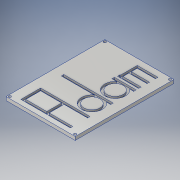
# Autodesk Inventor part: Adam Name Plate
Saved by Autodesk Inventor 2016 (Build 200138000, 138)
## iProperties
Created: 2016-09-22
Part Number: Adam Name Plate
Material: Aluminum
Document SubType Name: Modeling
Designer: Adam Popescu
Density: 2.7 g/cm^3
Appearance: Aluminum - Flat
Sheet Metal Rule: Default
Author: Adam Popescu
Autodesk Inventor part; units mm, degrees
ref_plane "YZ Plane" through (0, 0, 0) normal (1, 0, 0) x (0, 1, 0)
ref_plane "XZ Plane" through (0, 0, 0) normal (0, 1, 0) x (-1, 0, 0)
ref_plane "XY Plane" through (0, 0, 0) normal (0, 0, 1) x (1, 0, 0)
sketch "Sketch1" plane through (0, 0, 0) normal (0, 1, 0) x (-1, 0, 0)
  line L0 (121.4597, 127.3409) -> (-56.3403, 127.3409)
  line L1 (-56.3403, 127.3409) -> (-56.3403, -126.6591)
  line L2 (-56.3403, -126.6591) -> (121.4597, -126.6591)
  line L3 (121.4597, -126.6591) -> (121.4597, 127.3409)
  point P0 (0, 0)
  dimension "d0" = 254
  dimension "d1" = 177.8
  constraints: 8 end point, 2 parallel, 1 horizontal, 1 perpendicular
  measures "d0" distance of L2.end L0.start
  measures "d1" distance of L0.start L0.end
sketch "Sketch2" plane through (0, 0, 0) normal (0, 1, 0) x (-1, 0, 0)
  point P0 (0, 0)
extrude "Extrusion1" add sketch "Sketch1" along normal blind 8.89
sketch "Sketch3" plane through (0, 8.89, 0) normal (0, 1, 0) x (1, 0, 0)
  line L0 (30.9403, -114.6409) -> (30.9403, -108.2909)
  line L1 (-121.4597, -127.3409) -> (56.3403, -127.3409) projected
  line L2 (56.3403, -127.3409) -> (56.3403, 126.6591) projected
  line L3 (30.9403, -108.2909) -> (-96.0597, -108.2909)
  line L4 (-96.0597, -108.2909) -> (-96.0597, -114.6409)
  line L5 (-96.0597, -114.6409) -> (30.9403, -114.6409)
  line L6 (-121.4597, 126.6591) -> (-121.4597, -127.3409) projected
  line L7 (-96.0597, -108.2909) -> (-89.7097, -108.2909)
  line L8 (-89.7097, -108.2909) -> (-89.7097, -63.8409)
  line L9 (-89.7097, -63.8409) -> (-96.0597, -63.8409)
  line L10 (-96.0597, -63.8409) -> (-96.0597, -108.2909)
  line L11 (-96.0597, -63.8409) -> (30.9403, -63.8409)
  line L12 (30.9403, -63.8409) -> (30.9403, -70.1909)
  line L13 (30.9403, -70.1909) -> (-96.0597, -70.1909)
  line L14 (-96.0597, -70.1909) -> (-96.0597, -63.8409)
  line L15 (-35.7347, -114.6409) -> (-29.3847, -114.6409)
  line L16 (-29.3847, -114.6409) -> (-29.3847, -63.8409)
  line L17 (-29.3847, -63.8409) -> (-35.7347, -63.8409)
  line L18 (-35.7347, -63.8409) -> (-35.7347, -114.6409)
  point P0 (0, 0)
  dimension "d4" = 6.35
  dimension "d5" = 12.7
  dimension "d6" = 25.4
  dimension "d7" = 25.4
  dimension "d8" = 6.35
  dimension "d10" = 127
  dimension "d11" = 6.35
  dimension "d12" = 50.8
  dimension "d13" = 6.35
  dimension "d14" = 60.325
  dimension "d15" = 60.325
  constraints: 32 end point, 6 parallel, 5 perpendicular, 4 horizontal, 2 point on line, 1 vertical
  measures "d4" distance of L0.start L0.end
  measures "d5" distance from line of L1 L0.start
  measures "d6" distance between parallel lines of L2 L0
  measures "d7" distance between parallel lines of L4 L6
  measures "d8" distance of L8.end L9.end
  measures "d10" distance of L9.end L11.end
  measures "d11" distance between parallel lines of L11 L13
  measures "d12" distance between parallel lines of L9 L5
  measures "d13" distance between parallel lines of L16 L18
  measures "d14" distance between parallel lines of L10 L18
  measures "d15" distance between parallel lines of L0 L16
sketch "Sketch4" plane through (0, 8.89, 0) normal (0, 1, 0) x (1, 0, 0)
  point P0 (0, 0)
extrude "Extrusion2" cut sketch "Sketch3" against normal blind 5.08 contours L5 L16 L3 L0 | L5 L18 L3 L16 | L3 L18 L13 L16 | L5 L4 L3 L18 | L16 L11 L12 L13 | L13 L18 L11 L16 | L3 L10 L13 L8 | L13 L8 L11 L18 | L13 L10 L9 L8
sketch "Sketch5" plane through (0, 8.89, 0) normal (0, 1, 0) x (1, 0, 0)
  line L0 (-96.0597, -4.1509) -> (30.9403, -4.1509)
  line L1 (30.9403, -4.1509) -> (30.9403, -10.5009)
  line L2 (30.9403, -10.5009) -> (-96.0597, -10.5009)
  line L3 (-96.0597, -10.5009) -> (-96.0597, -4.1509)
  line L4 (-96.0597, -63.8409) -> (30.9403, -63.8409) projected
  line L5 (-121.4597, 126.6591) -> (-121.4597, -127.3409) projected
  circle A0 centre (4.1687, -32.0909) radius 20.4377
  circle A1 centre (4.1687, -32.0909) radius 26.7877
  line L6 (56.3403, -127.3409) -> (56.3403, 126.6591) projected
  point P0 (0, 0)
  dimension "d18" = 53.34
  dimension "d19" = 6.35
  dimension "d20" = 127
  dimension "d21" = 25.4
  dimension "d22" = 6.35
  dimension "d23" = 21.59
  dimension "d24" = 100.2284
  dimension "d25" = 52.1716
  constraints: 8 end point, 2 centre point, 2 parallel, 1 coincident, 1 horizontal, 1 perpendicular
  measures "d18" distance between parallel lines of L4 L2
  measures "d19" distance of L2.end L0.start
  measures "d20" distance of L1.end L2.end
  measures "d21" distance between parallel lines of L5 L3
  measures "d22" radial gap between concentric circles of A1 A0
  measures "d23" distance from line of L2 A1.centre
  measures "d24" distance from line of L3 A1.centre
  measures "d25" distance from line of L6 A1.centre
sketch "Sketch6" plane through (0, 8.89, 0) normal (0, 1, 0) x (1, 0, 0)
  point P0 (0, 0)
extrude "Extrusion3" cut sketch "Sketch5" against normal blind 5.08
sketch "Sketch7" plane through (0, 8.89, 0) normal (0, 1, 0) x (1, 0, 0)
  line L0 (30.9403, 55.5391) -> (-32.5597, 55.5391)
  line L1 (-32.5597, 55.5391) -> (-32.5597, 48.0334)
  line L2 (-32.5597, 48.0334) -> (30.9403, 48.0334)
  line L3 (30.9403, 48.0334) -> (30.9403, 55.5391)
  line L4 (56.3403, -127.3409) -> (56.3403, 126.6591) projected
  line L5 (30.9403, -4.1509) -> (30.9403, -10.5009) projected
  circle A0 centre (4.1687, 27.5991) radius 20.4343
  circle A1 centre (4.1687, 27.5991) radius 26.7843
  line L6 (-96.0597, -4.1509) -> (30.9403, -4.1509) projected
  line L7 (-96.0597, -63.8409) -> (30.9403, -63.8409) projected
  arc A2 (-11.6885, -10.5009) -> (20.0259, -10.5009) centre (4.1687, -32.0909) ccw projected
  point P0 (0, 0)
  dimension "d31" = 25.4
  dimension "d35" = 31.75
  dimension "d37" = 27.94
  dimension "d39" = 27.94
  dimension "d40" = 63.5
  dimension "d42" = 25.4
  dimension "d43" = 26.7716
  dimension "d44" = 26.7716
  dimension "d45" = 31.75
  dimension "d46" = 6.35
  constraints: 8 end point, 2 centre point, 2 parallel, 1 coincident, 1 horizontal, 1 perpendicular, 1 tangent
  measures "d31" distance between parallel lines of L4 L5
  measures "d35" distance from line of L7 A2.centre
  measures "d37" distance from line of L6 A2.centre
  measures "d39" distance from line of L0 A0.centre
  measures "d40" distance between parallel lines of L3 L1
  measures "d42" distance between parallel lines of L4 L3
  measures "d43" distance from line of L3 A0.centre
  measures "d44" distance from line of L5 A2.centre
  measures "d45" distance from line of L6 A0.centre
  measures "d46" radial gap between concentric circles of A0 A1
sketch "Sketch9" plane through (0, 8.89, 0) normal (0, 1, 0) x (1, 0, 0)
  point P0 (0, 0)
extrude "Extrusion4" cut sketch "Sketch7" against normal blind 5.08 contours A1 L2 | L2 A1
sketch "Sketch12" plane through (0, 8.89, 0) normal (0, 1, 0) x (1, 0, 0)
  point P0 (0, 0)
sketch "Sketch13" plane through (0, 8.89, 0) normal (0, 1, 0) x (1, 0, 0)
  line L0 (30.9403, 48.4271) -> (-24.9397, 48.4271)
  line L1 (-24.9397, 48.4271) -> (-24.9397, 54.7771)
  line L2 (-24.9397, 54.7771) -> (30.9403, 54.7771)
  line L3 (30.9403, 54.7771) -> (30.9403, 48.4271)
  line L4 (56.3403, -127.3409) -> (56.3403, 126.6591) projected
  line L5 (-96.0597, -4.1509) -> (30.9403, -4.1509) projected
  point P0 (0, 0)
  dimension "d53" = 6.35
  dimension "d54" = 25.4
  dimension "d55" = 55.88
  dimension "d56" = 52.578
  constraints: 8 end point, 2 parallel, 1 horizontal, 1 perpendicular
  measures "d53" distance of L0.end L1.end
  measures "d54" distance between parallel lines of L4 L3
  measures "d55" distance of L0.start L0.end
  measures "d56" distance between parallel lines of L5 L0
extrude "Extrusion5" cut sketch "Sketch13" against normal blind 5.08
sketch "Sketch15" plane through (0, 8.89, 0) normal (0, 1, 0) x (1, 0, 0)
  point P0 (0, 0)
sketch "Sketch16" plane through (0, 8.89, 0) normal (0, 1, 0) x (1, 0, 0)
  point P0 (0, 0)
sketch "Sketch14" plane through (0, 8.89, 0) normal (0, 1, 0) x (1, 0, 0)
  line L0 (30.9403, 61.1271) -> (-23.4198, 61.1271)
  line L1 (-23.4198, 61.1271) -> (-23.4198, 67.4771)
  line L2 (-23.4198, 67.4771) -> (30.9403, 67.4771)
  line L3 (30.9403, 67.4771) -> (30.9403, 61.1271)
  line L4 (-24.9397, 54.7771) -> (30.9403, 54.7771) projected
  line L5 (-22.0163, 67.4771) -> (-15.6663, 67.4771)
  line L6 (-15.6663, 67.4771) -> (-15.6663, 82.7171)
  line L7 (-15.6663, 82.7171) -> (-22.0163, 82.7171)
  line L8 (-22.0163, 82.7171) -> (-22.0163, 67.4771)
  line L9 (-22.0163, 82.7171) -> (30.9403, 82.7171)
  line L10 (30.9403, 82.7171) -> (30.9403, 89.0671)
  line L11 (30.9403, 89.0671) -> (-22.0163, 89.0671)
  line L12 (-22.0163, 89.0671) -> (-22.0163, 82.7171)
  line L13 (-22.0163, 89.0671) -> (-15.6663, 89.0671)
  line L14 (-15.6663, 89.0671) -> (-15.6663, 104.3071)
  line L15 (-15.6663, 104.3071) -> (-22.0163, 104.3071)
  line L16 (-22.0163, 104.3071) -> (-22.0163, 89.0671)
  line L17 (-22.0163, 104.3071) -> (30.9403, 104.3071)
  line L18 (30.9403, 104.3071) -> (30.9403, 110.6571)
  line L19 (30.9403, 110.6571) -> (-22.0163, 110.6571)
  line L20 (-22.0163, 110.6571) -> (-22.0163, 104.3071)
  point P0 (0, 0)
  dimension "d59" = 6.35
  dimension "d60" = 6.35
  dimension "d61" = 6.35
  dimension "d62" = 15.24
  dimension "d63" = 6.35
  dimension "d64" = 15.24
  dimension "d65" = 6.35
  dimension "d66" = 6.35
  constraints: 40 end point, 10 parallel, 5 horizontal, 5 perpendicular, 1 point on line
  measures "d59" distance between parallel lines of L4 L0
  measures "d60" distance between parallel lines of L2 L0
  measures "d61" distance between parallel lines of L6 L8
  measures "d62" distance of L7.end L5.start
  measures "d63" distance between parallel lines of L11 L9
  measures "d64" distance of L15.end L11.end
  measures "d65" distance of L14.end L15.end
  measures "d66" distance of L17.end L18.end
extrude "Extrusion6" cut sketch "Sketch14" against normal blind 5.08
sketch "Sketch19" plane through (0, 3.81, 0) normal (0, 1, 0) x (1, 0, 0)
  point P0 (0, 0)
sketch "Sketch21" plane through (0, 8.89, 0) normal (0, 1, 0) x (1, 0, 0)
  circle A0 centre (-116.3797, -122.2609) radius 3.175
  line L0 (-121.4597, 126.6591) -> (-121.4597, -127.3409) projected
  line L1 (-121.4597, -127.3409) -> (56.3403, -127.3409) projected
  point P0 (0, 0)
  dimension "d69" = 6.35
  dimension "d70" = 5.08
  dimension "d71" = 5.08
  constraints: 1 centre point
  measures "d69" diameter of A0
  measures "d70" distance from line of L0 A0.centre
  measures "d71" distance from line of L1 A0.centre
sketch "Sketch22" plane through (0, 8.89, 0) normal (0, 1, 0) x (1, 0, 0)
  circle A0 centre (51.2603, -122.2609) radius 3.175
  line L0 (56.3403, -127.3409) -> (56.3403, 126.6591) projected
  line L1 (-121.4597, -127.3409) -> (56.3403, -127.3409) projected
  circle A1 centre (-116.3797, 121.5791) radius 3.175
  line L2 (56.3403, 126.6591) -> (-121.4597, 126.6591) projected
  line L3 (-121.4597, 126.6591) -> (-121.4597, -127.3409) projected
  circle A2 centre (51.2603, 121.5791) radius 3.175
  point P0 (0, 0)
  dimension "d72" = 6.35
  dimension "d73" = 5.08
  dimension "d74" = 5.08
  dimension "d75" = 6.35
  dimension "d76" = 5.08
  dimension "d77" = 5.08
  dimension "d78" = 6.35
  dimension "d79" = 5.08
  dimension "d80" = 5.08
  constraints: 3 centre point
  measures "d72" diameter of A0
  measures "d73" distance from line of L0 A0.centre
  measures "d74" distance from line of L1 A0.centre
  measures "d75" diameter of A1
  measures "d76" distance from line of L2 A1.centre
  measures "d77" distance from line of L3 A1.centre
  measures "d78" diameter of A2
  measures "d79" distance from line of L0 A2.centre
  measures "d80" distance from line of L2 A2.centre
extrude "Extrusion7" cut sketch "Sketch22" against normal blind 25.4 contours A0 | A1 | A2
extrude "Extrusion8" cut sketch "Sketch21" against normal blind 25.4
equation "\"BendRadius\" = Thickness"
equation "\"BendReliefWidth\" = Thickness"
equation "\"BendReliefDepth\" = 0.5 * Thickness"
equation "\"CornerReliefSize\" = 4 * Thickness"
equation "\"MinimumRemnant\" = 2 * Thickness"
equation "\"TransitionRadius\" = BendRadius"
equation "\"JacobiRadiusSize\" = Thickness"
equation "\"GapSize\" = Thickness"
equation "\"Thickness\" = 3.048"
body "Solid1"
